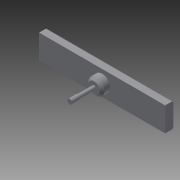
# Autodesk Inventor part: tempathook
Saved by Autodesk Inventor 2013 (Build 170138000, 138)
## iProperties
Created: 2016-04-12
Part Number: tempathook
Material: Generic
Document SubType Name: Modeling
Designer: yuyudhn
Density: 1 g/cm^3
Author: yuyudhn
Autodesk Inventor part; units mm, degrees
ref_plane "YZ Plane" through (0, 0, 0) normal (1, 0, 0) x (0, 1, 0)
ref_plane "XZ Plane" through (0, 0, 0) normal (0, 1, 0) x (-1, 0, 0)
ref_plane "XY Plane" through (0, 0, 0) normal (0, 0, 1) x (1, 0, 0)
sketch "Sketch1" plane through (0, 0, 0) normal (0, 1, 0) x (-1, 0, 0)
  line L0 (0, 0) -> (15580, 0)
  line L1 (15580, 0) -> (15580, -3000)
  line L2 (15580, -3000) -> (0, -3000)
  line L3 (0, -3000) -> (0, 0)
  dimension "d0" = 15580
  dimension "d1" = 3000
  constraints: 8 end point, 2 parallel, 1 horizontal, 1 perpendicular
  measures "d0" distance of L1.end L2.end
  measures "d1" distance of L0.end L1.end
extrude "Extrusion1" add sketch "Sketch1" along normal blind 1000
fillet "Fillet1" radius 200 2 edges at (-7790, 1000, 0) (-7790, 1000, -3000)
sketch "Sketch2" plane through (0, 0, 0) normal (0, -1, 0) x (1, 0, 0)
  circle A0 centre (-7790, -1500) radius 1000
  dimension "d5" = 2000
  constraints: 1 centre point
  measures "d5" diameter of A0
extrude "Extrusion2" add sketch "Sketch2" along normal blind 1000
sketch "Sketch3" plane through (-7790, -1000, -1500) normal (0, -1, 0) x (1, 0, 0)
  circle A0 centre (0, 0) radius 1000 projected
  circle A1 centre (0, 0) radius 250
  point P0 (7790, 1500)
  dimension "d8" = 500
  constraints: 1 centre point, 1 coincident
  measures "d8" diameter of A1
extrude "Extrusion3" add sketch "Sketch3" along normal blind 2000 contours A1
sketch "Sketch4" plane through (-7790, -3000, -1500) normal (0, -1, 0) x (1, 0, 0)
  circle A0 centre (0, 0) radius 250 projected
  circle A1 centre (0, 0) radius 300
  point P0 (7790, 1500)
  dimension "d12" = 600
  constraints: 1 centre point, 1 coincident
  measures "d12" diameter of A1
extrude "Extrusion4" add sketch "Sketch4" along normal blind 1000 contours A0 | A1
sketch "Sketch5" plane through (-7790, -4000, -1500) normal (0, -1, 0) x (1, 0, 0)
  circle A0 centre (0, 0) radius 300 projected
  circle A1 centre (0, 0) radius 50
  point P0 (7790, 1500)
  dimension "d15" = 100
  constraints: 1 centre point, 1 coincident
  measures "d15" diameter of A1
extrude "Extrusion5" cut sketch "Sketch5" against normal blind 500 contours A1
thread "Thread1" size "M100x6" class "6H" standard "ANSI Metric M Profile" full length
chamfer "Chamfer1" distance 30 angle 45 1 edges at (-8090, -3000, -1500)
chamfer "Chamfer2" distance 300 angle 45 1 edges at (-8790, -1000, -1500)
body "Solid1"
